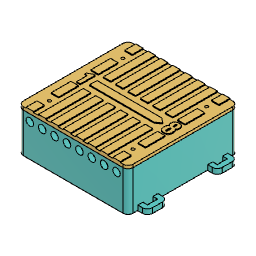
RelayBox (Autodesk Fusion 360 design; units mm, degrees)
Autodesk Fusion 360 part; units mm, degrees
(part 1 of 2)
sketch "Skizze1" plane through (0, 0, 0) normal (0, 0, 1) x (1, 0, 0)
  line L0 (0, 0) -> (110, 0)
  line L1 (110, 0) -> (110, 110)
  line L2 (110, 110) -> (0, 110)
  line L3 (0, 110) -> (0, 0)
  dimension "d1" = 110
  dimension "d2" = 110
  constraint horizontal L0
  constraint vertical L1
  constraint horizontal L2
  constraint vertical L3
  constraint coincident L0.start L3.end
  measures "d1" distance of L0.start L0.end
  measures "d2" distance of L0.start L2.end
extrude "Extrusion1" add sketch "Skizze1" along normal blind 40 makes body 1
sketch "Skizze2" plane through (0, 0, 0) normal (0, -1, 0) x (1, 0, 0)
  line L0 (0, 0) -> (110, 0)
  line L1 (110, 0) -> (110, 40)
  line L2 (110, 40) -> (0, 40)
  line L3 (0, 40) -> (0, 0)
  line L4 (0, 33) -> (110, 33)
  circle A0 centre (11.5, 33) radius 3.75
  circle A1 centre (11.5, 33) radius 5.5 construction
  circle A2 centre (-1832.7857, 33) radius 3.75
  circle A3 centre (-1832.7857, 33) radius 5.5 construction
  circle A4 centre (-3677.0714, 33) radius 3.75
  circle A5 centre (-3677.0714, 33) radius 5.5 construction
  circle A6 centre (-5521.3571, 33) radius 3.75
  circle A7 centre (-5521.3571, 33) radius 5.5 construction
  circle A8 centre (-7365.6429, 33) radius 3.75
  circle A9 centre (-7365.6429, 33) radius 5.5 construction
  circle A10 centre (-9209.9286, 33) radius 3.75
  circle A11 centre (-9209.9286, 33) radius 5.5 construction
  circle A12 centre (-11054.2143, 33) radius 3.75
  circle A13 centre (-11054.2143, 33) radius 5.5 construction
  circle A14 centre (-12898.5, 33) radius 3.75
  circle A15 centre (-12898.5, 33) radius 5.5 construction
  circle A16 centre (23.9286, 33) radius 5.5 construction
  circle A17 centre (23.9286, 33) radius 3.75
  circle A18 centre (36.3571, 33) radius 5.5 construction
  circle A19 centre (36.3571, 33) radius 3.75
  circle A20 centre (48.7857, 33) radius 5.5 construction
  circle A21 centre (48.7857, 33) radius 3.75
  circle A22 centre (61.2143, 33) radius 5.5 construction
  circle A23 centre (61.2143, 33) radius 3.75
  circle A24 centre (73.6429, 33) radius 5.5 construction
  circle A25 centre (73.6429, 33) radius 3.75
  circle A26 centre (86.0714, 33) radius 5.5 construction
  circle A27 centre (86.0714, 33) radius 3.75
  circle A28 centre (98.5, 33) radius 5.5 construction
  circle A29 centre (98.5, 33) radius 3.75
  dimension "d5" = 33
  dimension "d7" = 110
  dimension "d8" = 7.5
  dimension "d9" = 11.5
  dimension "d12" = 11
  dimension "d15" = -12910
  dimension "d16" = 0
  dimension "d19" = 87
  dimension "d20" = 0
  constraint coincident L3 L4.start
  constraint coincident L1 L4.end
  constraint perpendicular L1 L4
  constraint coincident L4 A0.centre
  constraint concentric A0 A1
  measures "d5" distance of L0 L4
  measures "d7" distance of L1.end L2.end
  measures "d8" diameter of A0
  measures "d9" distance of L3 A0.centre
  measures "d12" diameter of A1
extrude "Extrusion2" cut sketch "Skizze2" against normal blind 110 contours L4 A0 | L4 A0 | L4 A29 | L4 A29 | L4 A17 | L4 A17 | L4 A27 | L4 A27 | L4 A19 | L4 A19 | L4 A25 | L4 A25 | L4 A21 | L4 A21 | L4 A23 | L4 A23 bodies 1
sketch "Skizze3" plane through (0, 0, 40) normal (0, 0, 1) x (-1, 0, 0)
  line L0 (0, -110) -> (0, 0)
  line L1 (0, 0) -> (-110, 0)
  line L2 (-110, 0) -> (-110, -110)
  line L3 (-110, -110) -> (0, -110)
  line L4 (-105, -105) -> (-5, -105)
  line L5 (-5, -105) -> (-5, -5)
  line L6 (-5, -5) -> (-105, -5)
  line L7 (-105, -5) -> (-105, -105)
  dimension "d23" = -5
extrude "Extrusion3" cut sketch "Skizze3" against normal blind 35 contours L4 L5 L6 L7 bodies 1
sketch "Skizze4" plane through (0, 0, 5) normal (0, 0, 1) x (-1, 0, 0)
  line L0 (-105, -5) -> (-105, -105)
  line L1 (-105, -105) -> (-5, -105)
  line L2 (-5, -105) -> (-5, -5)
  line L3 (-5, -5) -> (-105, -5)
  line L4 (-100.75, -95.1) -> (-9.25, -95.1)
  line L5 (-9.25, -95.1) -> (-9.25, -14.9)
  line L6 (-9.25, -14.9) -> (-100.75, -14.9)
  line L7 (-100.75, -14.9) -> (-100.75, -95.1)
  dimension "d26" = 80.2
  dimension "d27" = 91.5
  dimension "d28" = 100
  dimension "d29" = 9.9
  dimension "d30" = 100
  dimension "d31" = 4.25
  constraint horizontal L4
  constraint vertical L5
  constraint horizontal L6
  constraint vertical L7
  measures "d26" distance of L4.start L6.end
  measures "d27" distance of L5.end L6.end
  measures "d28" distance of L1.end L2.end
  measures "d29" distance of L3 L6
  measures "d30" distance of L0.end L1.end
  measures "d31" distance of L0 L7
sketch "Skizze5" plane through (0, 0, 5) normal (0, 0, 1) x (-1, 0, 0)
  line L0 (-13.05, -18.1) -> (-13.05, -91.9)
  line L1 (-13.05, -91.9) -> (-96.95, -91.9)
  line L2 (-96.95, -91.9) -> (-96.95, -18.1)
  line L3 (-13.05, -18.1) -> (-96.95, -18.1)
  line L4 (0, 0) -> (-110, 0)
  line L5 (-5, -105) -> (-105, -105)
  line L6 (-105, -105) -> (-105, -5)
  line L7 (-105, -5) -> (-5, -5)
  line L8 (-5, -5) -> (-5, -105)
  line L9 (0, -110) -> (0, 0)
  line L10 (0, 0) -> (-110, 0)
  line L11 (-110, 0) -> (-110, -110)
  line L12 (-110, -110) -> (0, -110)
  line L13 (-55, 0) -> (-55, -110)
  line L14 (-110, -55) -> (0, -55)
  circle A0 centre (-96.95, -18.1) radius 2.5
  circle A1 centre (-96.95, -18.1) radius 5
  circle A2 centre (-13.05, -18.1) radius 2.5
  circle A3 centre (-13.05, -91.9) radius 2.5
  circle A4 centre (-96.95, -91.9) radius 2.5
  circle A5 centre (-96.95, -91.9) radius 5
  circle A6 centre (-13.05, -91.9) radius 5
  circle A7 centre (-13.05, -18.1) radius 5
  dimension "d32" = 73.8
  dimension "d33" = 83.9
  dimension "d34" = 73.8
  dimension "d35" = 5
  dimension "d36" = 10
  dimension "d37" = 5
  dimension "d38" = 5
  dimension "d39" = 5
  dimension "d40" = 10
  dimension "d41" = 10
  dimension "d42" = 10
  constraint vertical L0
  constraint perpendicular L0 L1
  constraint perpendicular L1 L2
  constraint midpoint L4 L13.start
  constraint midpoint L12 L13.end
  constraint midpoint L11 L14.start
  constraint midpoint L9 L14.end
  constraint symmetric L1 L3 L14
  constraint coincident L2.end L3.end
  constraint concentric A0 A1
  constraint coincident L0.start L3.start
  constraint coincident L0.end L1.start
  constraint coincident L1.end L2.start
  constraint concentric A4 A5
  constraint concentric A3 A6
  constraint concentric A2 A7
  measures "d32" distance of L0.start L0.end
  measures "d33" distance of L0.end L1.end
  measures "d34" distance of L1.end L2.end
  measures "d35" diameter of A0
  measures "d36" diameter of A1
  measures "d37" diameter of A2
  measures "d38" diameter of A3
  measures "d39" diameter of A4
  measures "d40" diameter of A5
  measures "d41" diameter of A6
  measures "d42" diameter of A7
extrude "Extrusion4" add sketch "Skizze5" along normal blind 3 contours L0 L3 A2 A7 | L0 L3 A2 A7 | L0 L1 A3 A6 | L0 L1 A3 A6 | L2 L3 A0 A1 | L2 L3 A0 A1 | L1 L2 A4 A5 | L1 L2 A4 A5 bodies 1
sketch "Skizze6" plane through (0, 0, 8) normal (0, 0, 1) x (-1, 0, 0)
  circle A0 centre (-96.95, -18.1) radius 2.5
  circle A1 centre (-96.95, -18.1) radius 5
  circle A2 centre (-96.95, -91.9) radius 2.5
  circle A3 centre (-96.95, -18.1) radius 2.5
  circle A4 centre (-13.05, -18.1) radius 2.5
  circle A5 centre (-13.05, -91.9) radius 2.5
  circle A6 centre (-13.05, -18.1) radius 2.5
extrude "Extrusion5" cut sketch "Skizze6" against normal blind 6 contours A0 A3 | A2 | A4 A6 | A5 bodies 1
sketch "Skizze7" plane through (0, 110, 0) normal (0, 1, 0) x (-1, 0, 0)
  circle A0 centre (-73.6429, 33) radius 3.75
  circle A1 centre (-23.9286, 33) radius 3.75
  circle A2 centre (-36.3571, 33) radius 3.75
  circle A3 centre (-86.0714, 33) radius 3.75
  circle A4 centre (-61.2143, 33) radius 3.75
  circle A5 centre (-11.5, 33) radius 3.75
  circle A6 centre (-48.7857, 33) radius 3.75
  circle A7 centre (-98.5, 33) radius 3.75
  line L0 (-110, 0) -> (0, 0)
  line L1 (0, 0) -> (0, 40)
  line L2 (0, 40) -> (-110, 40)
  line L3 (-110, 40) -> (-110, 0)
  line L4 (-99.45, 8) -> (-94.45, 8)
  line L5 (-15.55, 8) -> (-10.55, 8)
  line L6 (-94.45, 8) -> (-53.45, 8)
  line L7 (-15.55, 8) -> (-42.55, 8)
  line L8 (-53.45, 8) -> (-53.45, 14)
  line L9 (-42.55, 8) -> (-42.55, 14)
  line L10 (-42.55, 14) -> (-53.45, 14)
  line L11 (-53.45, 8) -> (-42.55, 8)
  dimension "d47" = 41
  dimension "d48" = 27
  dimension "d49" = 6
  dimension "d50" = 6
  constraint coincident L4.end L6.start
  constraint parallel L4 L6
  constraint coincident L5.start L7.start
  constraint parallel L5 L7
  constraint perpendicular L6 L8
  constraint perpendicular L7 L9
  measures "d47" distance of L4.end L6.end
  measures "d48" distance of L5.start L7.end
  measures "d49" distance of L6.end L8.end
  measures "d50" distance of L7.end L9.end
extrude "Extrusion6" cut sketch "Skizze7" against normal blind 5 contours L8 L9 L10 L11 bodies 1
sketch "Skizze8" plane through (0, 110, 0) normal (0, 1, 0) x (-1, 0, 0)
  line L0 (-42.55, 14) -> (-42.55, 8)
  line L1 (-42.55, 8) -> (-53.45, 8)
  line L2 (-53.45, 8) -> (-53.45, 14)
  line L3 (-53.45, 14) -> (-42.55, 14)
  circle A0 centre (-73.6429, 33) radius 3.75
  circle A1 centre (-23.9286, 33) radius 3.75
  circle A2 centre (-36.3571, 33) radius 3.75
  circle A3 centre (-86.0714, 33) radius 3.75
  circle A4 centre (-61.2143, 33) radius 3.75
  circle A5 centre (-11.5, 33) radius 3.75
  circle A6 centre (-48.7857, 33) radius 3.75
  circle A7 centre (-98.5, 33) radius 3.75
  line L4 (-110, 0) -> (0, 0)
  line L5 (0, 0) -> (0, 40)
  line L6 (0, 40) -> (-110, 40)
  line L7 (-110, 40) -> (-110, 0)
  circle A8 centre (-42.55, 11) radius 3
  circle A9 centre (-53.45, 11) radius 3
  constraint coincident L0.end A8
  constraint tangent L1 A8
  constraint coincident L0.start A8
  constraint coincident L1.end A9
  constraint tangent L1 A9
  constraint coincident L2.end A9
extrude "Extrusion7" cut sketch "Skizze8" against normal blind 5 contours L0 A8 | L2 A9 picked at (-41.5602, 11.1423) picked at (-54.4249, 10.7775) bodies 1
fillet "Abrundung1" radius 1 4 edges at (48, 110, 8) (56.45, 110, 11) (48, 110, 14) (39.55, 110, 11) on bodies 1
fillet "Abrundung2" radius 5 4 edges at (110, 110, 20) (110, 0, 20) (0, 0, 20) (0, 110, 20) on bodies 1
chamfer "Fase1" distance 0.4 angle 45 8 edges at (108.5355, 108.5355, 0) (55, 110, 0) (1.4645, 108.5355, 0) (0, 55, 0) (1.4645, 1.4645, 0) (55, 0, 0) (108.5355, 1.4645, 0) (110, 55, 0) on bodies 1
sketch "Skizze9" plane through (0, 0, 0) normal (0, 0, -1) x (1, 0, 0)
  arc A0 (105, -109.6) -> (109.6, -105) centre (105, -105) ccw
  line L0 (109.6, -105) -> (109.6, -5)
  arc A1 (109.6, -5) -> (105, -0.4) centre (105, -5) ccw
  line L1 (105, -0.4) -> (5, -0.4)
  arc A2 (5, -0.4) -> (0.4, -5) centre (5, -5) ccw
  line L2 (0.4, -5) -> (0.4, -105)
  arc A3 (0.4, -105) -> (5, -109.6) centre (5, -105) ccw
  line L3 (5, -109.6) -> (105, -109.6)
  line L4 (109.6, -95) -> (114.6, -95)
  line L5 (114.6, -95) -> (114.6, -85)
  line L6 (114.6, -85) -> (109.6, -85)
  line L7 (109.6, -85) -> (109.6, -95)
  line L8 (104.6, -100) -> (119.6, -100)
  line L9 (119.6, -100) -> (119.6, -80)
  line L10 (119.6, -80) -> (104.6, -80)
  line L11 (104.6, -80) -> (104.6, -100)
  line L12 (114.6, -15) -> (109.6, -15)
  line L13 (109.6, -15) -> (109.6, -25)
  line L14 (109.6, -25) -> (114.6, -25)
  line L15 (114.6, -25) -> (114.6, -15)
  line L16 (0.4, -15) -> (-4.6, -15)
  line L17 (-4.6, -15) -> (-4.6, -25)
  line L18 (-4.6, -25) -> (0.4, -25)
  line L19 (0.4, -25) -> (0.4, -15)
  line L20 (0.4, -85) -> (-4.6, -85)
  line L21 (-4.6, -85) -> (-4.6, -95)
  line L22 (-4.6, -95) -> (0.4, -95)
  line L23 (0.4, -95) -> (0.4, -85)
  line L24 (5, -110) -> (105, -110)
  line L25 (5.4, -100) -> (5.4, -80)
  line L26 (5.4, -80) -> (-9.6, -80)
  line L27 (-9.6, -80) -> (-9.6, -100)
  line L28 (-9.6, -100) -> (5.4, -100)
  line L29 (5.4, -30) -> (5.4, -10)
  line L30 (5.4, -10) -> (-9.6, -10)
  line L31 (-9.6, -10) -> (-9.6, -30)
  line L32 (-9.6, -30) -> (5.4, -30)
  line L33 (104.6, -30) -> (119.6, -30)
  line L34 (119.6, -30) -> (119.6, -10)
  line L35 (119.6, -10) -> (104.6, -10)
  line L36 (104.6, -10) -> (104.6, -30)
  line L37 (105, 0) -> (5, 0)
  dimension "d60" = 5
  dimension "d61" = 10
  dimension "d62" = 5
  dimension "d66" = 5
  dimension "d67" = 5
  dimension "d68" = 5
  dimension "d69" = 10
  dimension "d70" = 10
  dimension "d71" = 10
  dimension "d72" = 10
  dimension "d73" = 5
  dimension "d74" = 5
  dimension "d75" = 5
  dimension "d76" = 10
  dimension "d77" = 10
  dimension "d78" = 10
  constraint horizontal L4
  constraint vertical L5
  constraint horizontal L6
  constraint vertical L7
  constraint coincident L0 L4.start
  constraint horizontal L12
  constraint vertical L13
  constraint horizontal L14
  constraint vertical L15
  constraint horizontal L16
  constraint vertical L17
  constraint horizontal L18
  constraint vertical L19
  constraint horizontal L20
  constraint vertical L21
  constraint horizontal L22
  constraint vertical L23
  constraint collinear L2 L23
  constraint collinear L2 L19
  constraint collinear L0 L13
  constraint collinear L4 L22
  measures "d60" distance of L4.start L4.end
  measures "d61" distance of L4.start L6.end
  measures "d62" distance of L4
  measures "d66" distance of L21.end L22.end
  measures "d67" distance of L17.end L18.end
  measures "d68" distance of L13.end L14.end
  measures "d69" distance of L12.start L14.end
  measures "d70" distance of L16.end L17.end
  measures "d71" distance of L20.end L21.end
  measures "d72" distance of L8 L24
  measures "d75" distance of L14
  measures "d76" distance of L35 L37
  measures "d77" distance of L30 L37
  measures "d78" distance of L24 L28
extrude "Extrusion8" add sketch "Skizze9" against normal blind 5 contours L0 L4 L5 L6 L8 L9 L10 bodies 1
extrude "Extrusion9" add sketch "Skizze9" against normal blind 5 contours L2 L20 L21 L22 L26 L27 L28 | L0 L12 L14 L15 L33 L34 L35 | L2 L16 L17 L18 L30 L31 L32 bodies 1
fillet "Abrundung3" radius 5 8 edges at (119.6, 10, 2.5) (-9.6, 10, 2.5) (119.6, 30, 2.5) (119.6, 100, 2.5) (119.6, 80, 2.5) (-9.6, 30, 2.5) (-9.6, 80, 2.5) (-9.6, 100, 2.5) on bodies 1
sketch "Skizze10" plane through (0, 0, 40) normal (0, 0, 1) x (-1, 0, 0)
  arc A0 (-5, -110) -> (0, -105) centre (-5, -105) ccw
  line L0 (0, -105) -> (0, -5)
  arc A1 (0, -5) -> (-5, 0) centre (-5, -5) ccw
  line L1 (-5, 0) -> (-105, 0)
  arc A2 (-105, 0) -> (-110, -5) centre (-105, -5) ccw
  line L2 (-110, -5) -> (-110, -105)
  arc A3 (-110, -105) -> (-105, -110) centre (-105, -105) ccw
  line L3 (-105, -110) -> (-5, -110)
  line L4 (-5, -105) -> (-105, -105)
  line L5 (-105, -105) -> (-105, -5)
  line L6 (-105, -5) -> (-5, -5)
  line L7 (-5, -5) -> (-5, -105)
  circle A4 centre (-13.05, -91.9) radius 2.5
  circle A5 centre (-13.05, -18.1) radius 2.5
  circle A6 centre (-96.95, -18.1) radius 2.5
  circle A7 centre (-96.95, -91.9) radius 2.5
  circle A8 centre (-96.95, -18.1) radius 2.5
  line L8 (-104, -6) -> (-6, -6)
  line L9 (-6, -6) -> (-6, -104)
  line L10 (-6, -104) -> (-104, -104)
  line L11 (-104, -104) -> (-104, -6)
  circle A9 centre (-13.05, -91.9) radius 1.5
  circle A10 centre (-13.05, -18.1) radius 1.5
  circle A11 centre (-96.95, -18.1) radius 1.5
  circle A12 centre (-96.95, -91.9) radius 1.5
  dimension "d83" = 1
  dimension "d86" = 3
  dimension "d87" = 3
  dimension "d88" = 3
  dimension "d89" = 3
  constraint concentric A4 A9
  constraint concentric A5 A10
  constraint concentric A6 A11
  constraint concentric A7 A12
  measures "d86" diameter of A9
  measures "d87" diameter of A10
  measures "d88" diameter of A11
  measures "d89" diameter of A12
extrude "Extrusion11" add sketch "Skizze10" against normal blind 1 separate body contours A4 | A5 | A6 A8 | A7 | L8 L9 L10 L11 makes body 2
sketch "Skizze12" plane through (0, 0, 40) normal (0, 0, 1) x (-1, 0, 0)
extrude "Extrusion12" add sketch "Skizze10" along normal blind 3 separate body contours A0 L0 A1 L1 A2 L2 A3 L3 | L4 L5 L6 L7 | L8 L9 L10 L11 makes body 3
combine "Kombinieren1" operation add target body 2 tool bodies 3
sketch "Skizze13" plane through (0, 0, 43) normal (0, 0, 1) x (-1, 0, 0)
  circle A0 centre (-96.95, -18.1) radius 2.5
  circle A1 centre (-13.05, -91.9) radius 2.5
  circle A2 centre (-96.95, -91.9) radius 2.5
  circle A3 centre (-13.05, -18.1) radius 2.5
  line L0 (-105, -110) -> (-5, -110)
  arc A4 (-5, -110) -> (0, -105) centre (-5, -105) ccw
  line L1 (0, -105) -> (0, -5)
  arc A5 (0, -5) -> (-5, 0) centre (-5, -5) ccw
  line L2 (-5, 0) -> (-105, 0)
  arc A6 (-105, 0) -> (-110, -5) centre (-105, -5) ccw
  line L3 (-110, -5) -> (-110, -105)
  arc A7 (-110, -105) -> (-105, -110) centre (-105, -105) ccw
  line L4 (-15.25, 0) -> (-7.75, 0)
  line L5 (-27.6786, 0) -> (-20.1786, 0)
  line L6 (-40.1071, 0) -> (-32.6071, 0)
  line L7 (-52.5357, 0) -> (-45.0357, 0)
  line L8 (-64.9643, 0) -> (-57.4643, 0)
  line L9 (-77.3929, 0) -> (-69.8929, 0)
  line L10 (-89.8214, 0) -> (-82.3214, 0)
  line L11 (-102.25, 0) -> (-94.75, 0)
  line L12 (-7.75, 0) -> (-15.25, 0)
  line L13 (-15.25, 0) -> (-15.25, -110)
  line L14 (-15.25, -110) -> (-7.75, -110)
  line L15 (-7.75, -110) -> (-7.75, 0)
  line L16 (-20.1786, 0) -> (-27.6786, 0)
  line L17 (-27.6786, 0) -> (-27.6786, -110)
  line L18 (-27.6786, -110) -> (-20.1786, -110)
  line L19 (-20.1786, -110) -> (-20.1786, 0)
  line L20 (-32.6071, 0) -> (-40.1071, 0)
  line L21 (-40.1071, 0) -> (-40.1071, -110)
  line L22 (-40.1071, -110) -> (-32.6071, -110)
  line L23 (-32.6071, -110) -> (-32.6071, 0)
  line L24 (-45.0357, 0) -> (-52.5357, 0)
  line L25 (-52.5357, 0) -> (-52.5357, -110)
  line L26 (-52.5357, -110) -> (-45.0357, -110)
  line L27 (-45.0357, -110) -> (-45.0357, 0)
  line L28 (-57.4643, 0) -> (-64.9643, 0)
  line L29 (-64.9643, 0) -> (-64.9643, -110)
  line L30 (-64.9643, -110) -> (-57.4643, -110)
  line L31 (-57.4643, -110) -> (-57.4643, 0)
  line L32 (-69.8929, 0) -> (-77.3929, 0)
  line L33 (-77.3929, 0) -> (-77.3929, -110)
  line L34 (-77.3929, -110) -> (-69.8929, -110)
  line L35 (-69.8929, -110) -> (-69.8929, 0)
  line L36 (-82.3214, 0) -> (-89.8214, 0)
  line L37 (-89.8214, 0) -> (-89.8214, -110)
  line L38 (-89.8214, -110) -> (-82.3214, -110)
  line L39 (-82.3214, -110) -> (-82.3214, 0)
  line L40 (-94.75, 0) -> (-102.25, 0)
  line L41 (-102.25, 0) -> (-102.25, -110)
  line L42 (-102.25, -110) -> (-94.75, -110)
  line L43 (-94.75, -110) -> (-94.75, 0)
  constraint horizontal L12
  constraint vertical L13
  constraint horizontal L14
  constraint vertical L15
  constraint coincident L0 L13.end
  constraint coincident L4.end L12.start
  constraint horizontal L16
  constraint vertical L17
  constraint horizontal L18
  constraint vertical L19
  constraint coincident L0 L17.end
  constraint coincident L5.end L16.start
  constraint perpendicular L20 L21
  constraint parallel L20 L22
  constraint parallel L21 L23
  constraint coincident L6.start L20.end
  constraint perpendicular L17 L20
  constraint coincident L6.end L20.start
  constraint perpendicular L24 L25
  constraint parallel L24 L26
  constraint parallel L25 L27
  constraint coincident L7.start L24.end
  constraint perpendicular L23 L24
  constraint coincident L7.end L24.start
  constraint perpendicular L28 L29
  constraint parallel L28 L30
  constraint parallel L29 L31
  constraint coincident L8.start L28.end
  constraint perpendicular L27 L28
  constraint coincident L8.end L28.start
  constraint perpendicular L32 L33
  constraint parallel L32 L34
  constraint parallel L33 L35
  constraint coincident L9.start L32.end
  constraint perpendicular L31 L32
  constraint coincident L9.end L32.start
  constraint perpendicular L36 L37
  constraint parallel L36 L38
  constraint parallel L37 L39
  constraint coincident L10.start L36.end
  constraint perpendicular L35 L36
  constraint coincident L10.end L36.start
  constraint perpendicular L40 L41
  constraint parallel L40 L42
  constraint parallel L41 L43
  constraint coincident L11.start L40.end
  constraint perpendicular L39 L40
  constraint coincident L11.end L40.start
extrude "Extrusion13" add sketch "Skizze13" along normal blind 0.9 contours A0 A2 L0 L2 L11 L40 L41 L42 L43 | L0 L2 L10 L36 L37 L38 L39 | L0 L2 L9 L32 L33 L34 L35 | L0 L2 L8 L28 L29 L30 L31 | L0 L2 L7 L24 L25 L26 L27 | L0 L2 L6 L20 L21 L22 L23 | L0 L2 L5 L16 L17 L18 L19 | A1 A3 L0 L2 L4 L12 L13 L14 L15 bodies 2
sketch "Skizze14" plane through (0, 0, 43.9) normal (0, 0, 1) x (-1, 0, 0)
  line L0 (-15.25, -93.0874) -> (-15.25, -110)
  line L1 (-15.25, -110) -> (-7.75, -110)
  line L2 (-7.75, -110) -> (-7.75, 0)
  line L3 (-7.75, 0) -> (-15.25, 0)
  line L4 (-15.25, 0) -> (-15.25, -16.9126)
  arc A0 (-15.25, -19.2874) -> (-15.25, -16.9126) centre (-13.05, -18.1) ccw
  line L5 (-15.25, -19.2874) -> (-15.25, -90.7126)
  arc A1 (-15.25, -93.0874) -> (-15.25, -90.7126) centre (-13.05, -91.9) ccw
  line L6 (-20.1786, -110) -> (-20.1786, 0)
  line L7 (-89.8214, 0) -> (-89.8214, -110)
  line L8 (-20.1786, -10.9715) -> (-5.9214, -10.9715)
  line L9 (-5.9214, -10.9715) -> (-5.9214, -25.2285)
  line L10 (-5.9214, -25.2285) -> (-20.1786, -25.2285)
  line L11 (-20.1786, -25.2285) -> (-20.1786, -10.9715)
  line L12 (-20.1786, -10.9715) -> (-5.9214, -25.2285) construction
  line L13 (-5.9214, -10.9715) -> (-20.1786, -25.2285) construction
  line L14 (-5.9214, -10.9715) -> (-107.1918, -10.9715)
  line L15 (-5.9214, -25.2285) -> (-107.1184, -25.2285)
  line L16 (-94.75, -16.9126) -> (-94.75, 0)
  line L17 (-94.75, 0) -> (-102.25, 0)
  line L18 (-102.25, 0) -> (-102.25, -110)
  line L19 (-102.25, -110) -> (-94.75, -110)
  line L20 (-94.75, -110) -> (-94.75, -93.0874)
  arc A2 (-94.75, -90.7126) -> (-94.75, -93.0874) centre (-96.95, -91.9) ccw
  line L21 (-94.75, -90.7126) -> (-94.75, -19.2874)
  arc A3 (-94.75, -16.9126) -> (-94.75, -19.2874) centre (-96.95, -18.1) ccw
  line L22 (-7.75, -99.0285) -> (-102.25, -99.0285)
  line L23 (-102.25, -84.7715) -> (-7.75, -84.7715)
  point P0 (-13.05, -18.1)
  point P1 (-13.05, -91.9)
  dimension "d96" = 14.257
  dimension "d97" = 14.257
  dimension "d98" = 7.1285
  constraint horizontal L8
  constraint perpendicular L8 L9
  constraint parallel L8 L10
  constraint parallel L9 L11
  constraint coincident L12 P0
  constraint coincident L13 P0
  constraint coincident P0 A0.centre
  constraint perpendicular L9 L14
  constraint perpendicular L2 L15
  constraint coincident L2 L22.start
  constraint coincident L18 L22.end
  constraint perpendicular L18 L22
  constraint coincident L18 L23.start
  constraint coincident L2 L23.end
  constraint perpendicular L2 L23
  measures "d96" distance of L8.end L9.end
  measures "d97" distance of L22 L23
  measures "d98" distance of L22 P1
extrude "Extrusion14" cut sketch "Skizze14" against normal blind 0.9 contours L0 L2 L5 A1 L22 L23 | L2 L4 A0 L5 L8 L10 L14 L15 | L18 L20 A2 L21 L22 L23 | L14 L15 L16 L18 L21 A3 bodies 2
sketch "Skizze15" plane through (0, 0, 43.9) normal (0, 0, 1) x (-1, 0, 0)
  line L0 (-7.75, -25.2285) -> (-15.25, -25.2285)
  line L1 (-15.25, -25.2285) -> (-15.25, -84.7715)
  line L2 (-15.25, -84.7715) -> (-7.75, -84.7715)
  line L3 (-7.75, -84.7715) -> (-7.75, -25.2285)
  line L4 (-7.75, -25.2285) -> (-7.75, -84.7715)
  line L5 (-7.75, -84.7715) -> (-15.25, -84.7715)
  line L6 (-15.25, -84.7715) -> (-15.25, -25.2285)
  line L7 (-15.25, -25.2285) -> (-7.75, -25.2285)
  line L8 (-7.75, -10.9715) -> (-15.25, -10.9715)
  line L9 (-15.25, -10.9715) -> (-15.25, 0)
  line L10 (-15.25, 0) -> (-20.1786, 0)
  line L11 (-20.1786, 0) -> (-20.1786, -110)
  line L12 (-20.1786, -110) -> (-15.25, -110)
  line L13 (-15.25, -110) -> (-15.25, -99.0285)
  line L14 (-15.25, -99.0285) -> (-7.75, -99.0285)
  line L15 (-7.75, -99.0285) -> (-7.75, -110)
  line L16 (-7.75, -110) -> (-5, -110)
  arc A0 (-5, -110) -> (0, -105) centre (-5, -105) ccw
  line L17 (0, -105) -> (0, -5)
  arc A1 (0, -5) -> (-5, 0) centre (-5, -5) ccw
  line L18 (-5, 0) -> (-7.75, 0)
  line L19 (-7.75, 0) -> (-7.75, -10.9715)
  circle A2 centre (-13.05, -18.1) radius 2.5
  circle A3 centre (-13.05, -91.9) radius 2.5
  line L20 (-102.25, -84.7715) -> (-102.25, -25.2285)
  line L21 (-102.25, -25.2285) -> (-94.75, -25.2285)
  line L22 (-94.75, -25.2285) -> (-94.75, -84.7715)
  line L23 (-94.75, -84.7715) -> (-102.25, -84.7715)
  circle A4 centre (-96.95, -91.9) radius 2.5
  circle A5 centre (-96.95, -18.1) radius 2.5
  line L24 (-102.25, -99.0285) -> (-94.75, -99.0285)
  line L25 (-94.75, -99.0285) -> (-94.75, -110)
  line L26 (-94.75, -110) -> (-89.8214, -110)
  line L27 (-89.8214, -110) -> (-89.8214, 0)
  line L28 (-89.8214, 0) -> (-94.75, 0)
  line L29 (-94.75, 0) -> (-94.75, -10.9715)
  line L30 (-94.75, -10.9715) -> (-102.25, -10.9715)
  line L31 (-102.25, -10.9715) -> (-102.25, 0)
  line L32 (-102.25, 0) -> (-105, 0)
  arc A6 (-105, 0) -> (-110, -5) centre (-105, -5) ccw
  line L33 (-110, -5) -> (-110, -105)
  arc A7 (-110, -105) -> (-105, -110) centre (-105, -105) ccw
  line L34 (-105, -110) -> (-102.25, -110)
  line L35 (-102.25, -110) -> (-102.25, -99.0285)
  line L36 (-7.75, -55) -> (-102.25, -55)
  line L37 (-108.5309, -45) -> (-1.4691, -45)
  line L38 (-1.4691, -45) -> (-1.4691, -65)
  line L39 (-1.4691, -65) -> (-108.5309, -65)
  line L40 (-108.5309, -65) -> (-108.5309, -45)
  line L41 (-108.5309, -45) -> (-1.4691, -65) construction
  line L42 (-1.4691, -45) -> (-108.5309, -65) construction
  point P0 (-55, -55)
  dimension "d101" = 20
  constraint midpoint L4 L36.start
  constraint midpoint L20 L36.end
  constraint horizontal L37
  constraint perpendicular L37 L38
  constraint parallel L37 L39
  constraint parallel L38 L40
  constraint coincident L41 P0
  constraint coincident L42 P0
  constraint midpoint L36 P0
  measures "d101" distance of L37.end L38.end
extrude "Extrusion15" cut sketch "Skizze15" against normal blind 0.9 contours L1 L3 L4 L6 L36 L37 | L1 L3 L4 L6 L36 L39 | L11 L27 L36 L37 | L11 L27 L36 L39 | L20 L22 L36 L37 | L20 L22 L36 L39 bodies 2
sketch "Skizze16" plane through (0, 0, 43) normal (0, 0, 1) x (-1, 0, 0)
  line L0 (-102.25, -45) -> (-102.25, -25.2285)
  line L1 (-102.25, -25.2285) -> (-94.75, -25.2285)
  line L2 (-94.75, -25.2285) -> (-94.75, -45)
  line L3 (-94.75, -45) -> (-102.25, -45)
  circle A0 centre (-96.95, -18.1) radius 2.5
  circle A1 centre (-96.95, -91.9) radius 2.5
  line L4 (-102.25, -65) -> (-94.75, -65)
  line L5 (-94.75, -65) -> (-94.75, -84.7715)
  line L6 (-94.75, -84.7715) -> (-102.25, -84.7715)
  line L7 (-102.25, -84.7715) -> (-102.25, -65)
  line L8 (-7.75, -65) -> (-7.75, -84.7715)
  line L9 (-7.75, -84.7715) -> (-15.25, -84.7715)
  line L10 (-15.25, -84.7715) -> (-15.25, -65)
  line L11 (-15.25, -65) -> (-7.75, -65)
  line L12 (-7.75, -45) -> (-15.25, -45)
  line L13 (-15.25, -45) -> (-15.25, -25.2285)
  line L14 (-15.25, -25.2285) -> (-7.75, -25.2285)
  line L15 (-7.75, -25.2285) -> (-7.75, -45)
  line L16 (-7.75, -10.9715) -> (-15.25, -10.9715)
  line L17 (-15.25, -10.9715) -> (-15.25, 0)
  line L18 (-15.25, 0) -> (-20.1786, 0)
  line L19 (-20.1786, 0) -> (-20.1786, -45)
  line L20 (-20.1786, -45) -> (-27.6786, -45)
  line L21 (-27.6786, -45) -> (-27.6786, 0)
  line L22 (-27.6786, 0) -> (-32.6071, 0)
  line L23 (-32.6071, 0) -> (-32.6071, -45)
  line L24 (-32.6071, -45) -> (-40.1071, -45)
  line L25 (-40.1071, -45) -> (-40.1071, 0)
  line L26 (-40.1071, 0) -> (-45.0357, 0)
  line L27 (-45.0357, 0) -> (-45.0357, -45)
  line L28 (-45.0357, -45) -> (-52.5357, -45)
  line L29 (-52.5357, -45) -> (-52.5357, 0)
  line L30 (-52.5357, 0) -> (-57.4643, 0)
  line L31 (-57.4643, 0) -> (-57.4643, -45)
  line L32 (-57.4643, -45) -> (-64.9643, -45)
  line L33 (-64.9643, -45) -> (-64.9643, 0)
  line L34 (-64.9643, 0) -> (-69.8929, 0)
  line L35 (-69.8929, 0) -> (-69.8929, -45)
  line L36 (-69.8929, -45) -> (-77.3929, -45)
  line L37 (-77.3929, -45) -> (-77.3929, 0)
  line L38 (-77.3929, 0) -> (-82.3214, 0)
  line L39 (-82.3214, 0) -> (-82.3214, -45)
  line L40 (-82.3214, -45) -> (-89.8214, -45)
  line L41 (-89.8214, -45) -> (-89.8214, 0)
  line L42 (-89.8214, 0) -> (-94.75, 0)
  line L43 (-94.75, 0) -> (-94.75, -10.9715)
  line L44 (-94.75, -10.9715) -> (-102.25, -10.9715)
  line L45 (-102.25, -10.9715) -> (-102.25, 0)
  line L46 (-102.25, 0) -> (-105, 0)
  arc A2 (-105, 0) -> (-110, -5) centre (-105, -5) ccw
  line L47 (-110, -5) -> (-110, -105)
  arc A3 (-110, -105) -> (-105, -110) centre (-105, -105) ccw
  line L48 (-105, -110) -> (-102.25, -110)
  line L49 (-102.25, -110) -> (-102.25, -99.0285)
  line L50 (-102.25, -99.0285) -> (-94.75, -99.0285)
  line L51 (-94.75, -99.0285) -> (-94.75, -110)
  line L52 (-94.75, -110) -> (-89.8214, -110)
  line L53 (-89.8214, -110) -> (-89.8214, -65)
  line L54 (-89.8214, -65) -> (-82.3214, -65)
  line L55 (-82.3214, -65) -> (-82.3214, -110)
  line L56 (-82.3214, -110) -> (-77.3929, -110)
  line L57 (-77.3929, -110) -> (-77.3929, -65)
  line L58 (-77.3929, -65) -> (-69.8929, -65)
  line L59 (-69.8929, -65) -> (-69.8929, -110)
  line L60 (-69.8929, -110) -> (-64.9643, -110)
  line L61 (-64.9643, -110) -> (-64.9643, -65)
  line L62 (-64.9643, -65) -> (-57.4643, -65)
  line L63 (-57.4643, -65) -> (-57.4643, -110)
  line L64 (-57.4643, -110) -> (-52.5357, -110)
  line L65 (-52.5357, -110) -> (-52.5357, -65)
  line L66 (-52.5357, -65) -> (-45.0357, -65)
  line L67 (-45.0357, -65) -> (-45.0357, -110)
  line L68 (-45.0357, -110) -> (-40.1071, -110)
  line L69 (-40.1071, -110) -> (-40.1071, -65)
  line L70 (-40.1071, -65) -> (-32.6071, -65)
  line L71 (-32.6071, -65) -> (-32.6071, -110)
  line L72 (-32.6071, -110) -> (-27.6786, -110)
  line L73 (-27.6786, -110) -> (-27.6786, -65)
  line L74 (-27.6786, -65) -> (-20.1786, -65)
  line L75 (-20.1786, -65) -> (-20.1786, -110)
  line L76 (-20.1786, -110) -> (-15.25, -110)
  line L77 (-15.25, -110) -> (-15.25, -99.0285)
  line L78 (-15.25, -99.0285) -> (-7.75, -99.0285)
  line L79 (-7.75, -99.0285) -> (-7.75, -110)
  line L80 (-7.75, -110) -> (-5, -110)
  arc A4 (-5, -110) -> (0, -105) centre (-5, -105) ccw
  line L81 (0, -105) -> (0, -5)
  arc A5 (0, -5) -> (-5, 0) centre (-5, -5) ccw
  line L82 (-5, 0) -> (-7.75, 0)
  line L83 (-7.75, 0) -> (-7.75, -10.9715)
  circle A6 centre (-13.05, -18.1) radius 2.5
  circle A7 centre (-13.05, -91.9) radius 2.5
  line L84 (-17.7143, -45) -> (-5.2857, -45)
  line L85 (-5.2857, -45) -> (-5.2857, -65)
  line L86 (-5.2857, -65) -> (-17.7143, -65)
  line L87 (-17.7143, -65) -> (-17.7143, -45)
  line L88 (-30.1429, -65) -> (-30.1429, -45)
  line L89 (-17.7143, -65) -> (-30.1429, -65)
  line L90 (-17.7143, -45) -> (-17.7143, -65)
  line L91 (-30.1429, -45) -> (-17.7143, -45)
  line L92 (-42.5714, -65) -> (-42.5714, -45)
  line L93 (-30.1429, -65) -> (-42.5714, -65)
  line L94 (-30.1429, -45) -> (-30.1429, -65)
  line L95 (-42.5714, -45) -> (-30.1429, -45)
  line L96 (-55, -65) -> (-55, -45)
  line L97 (-42.5714, -65) -> (-55, -65)
  line L98 (-42.5714, -45) -> (-42.5714, -65)
  line L99 (-55, -45) -> (-42.5714, -45)
  line L100 (-67.4286, -65) -> (-67.4286, -45)
  line L101 (-55, -65) -> (-67.4286, -65)
  line L102 (-55, -45) -> (-55, -65)
  line L103 (-67.4286, -45) -> (-55, -45)
  line L104 (-79.8571, -65) -> (-79.8571, -45)
  line L105 (-67.4286, -65) -> (-79.8571, -65)
  line L106 (-67.4286, -45) -> (-67.4286, -65)
  line L107 (-79.8571, -45) -> (-67.4286, -45)
  line L108 (-92.2857, -65) -> (-92.2857, -45)
  line L109 (-79.8571, -65) -> (-92.2857, -65)
  line L110 (-79.8571, -45) -> (-79.8571, -65)
  line L111 (-92.2857, -45) -> (-79.8571, -45)
  line L112 (-104.7143, -65) -> (-104.7143, -45)
  line L113 (-92.2857, -65) -> (-104.7143, -65)
  line L114 (-92.2857, -45) -> (-92.2857, -65)
  line L115 (-104.7143, -45) -> (-92.2857, -45)
  line L116 (-5.2857, -45) -> (-17.7143, -45) construction
  line L117 (-17.7143, -45) -> (-17.7143, -65) construction
  line L118 (-17.7143, -65) -> (-5.2857, -65) construction
  line L119 (-5.2857, -65) -> (-5.2857, -45) construction
  line L120 (-92.2857, -45) -> (-104.7143, -45) construction
  line L121 (-104.7143, -45) -> (-104.7143, -65) construction
  line L122 (-104.7143, -65) -> (-92.2857, -65) construction
  line L123 (-92.2857, -65) -> (-92.2857, -45) construction
  dimension "d104" = 17.3571
  dimension "d105" = 4.9286
  dimension "d106" = 2.4643
  dimension "d107" = 2.4643
  dimension "d110" = -87
  dimension "d111" = 0
  dimension "d112" = 15
  dimension "d113" = 15
  text T0 "1" font "Impact" height 15 align centre middle in box 12.4286 x 20 at (-5.2857, -45) x (-1, 0) y (0, -1) spacing 1 kerned
  text T1 "8" font "Impact" height 15 align centre middle in box 12.4286 x 20 at (-92.2857, -45) x (-1, 0) y (0, -1) spacing 1 kerned
  constraint horizontal L84
  constraint vertical L85
  constraint horizontal L86
  constraint vertical L87
  constraint collinear L11 L86
  constraint collinear L20 L84
  constraint coincident L86.end
  constraint coincident L84.end
  constraint coincident L112.start
  constraint coincident L108.end
  measures "d104" distance of L12.end L23.end
  measures "d105" distance of L12.end L19.end
  measures "d106" distance of L13 L87
  measures "d107" distance of L15 L85
extrude "Extrusion16" add sketch "Skizze16" along normal blind 0.9 text T0 T1 bodies 2
sketch "Skizze17" plane through (0, 0, 43) normal (0, 0, 1) x (-1, 0, 0)
  spline S0 degree 3 poles (-101.2424, -56.0053) (-101.4993, -55.8834) (-101.9991, -55.6463) (-102.344, -55.2145) (-102.5117, -55.0046) knots 0 0 0 0 0.084034 0.16353 0.16353 0.16353 0.16353
  spline S1 degree 3 poles (-102.5117, -55.0046) (-102.6393, -54.6353) (-102.9898, -53.6205) (-102.9694, -52.5411) (-102.9565, -51.8545) knots 0 0 0 0 0.116519 0.320189 0.320189 0.320189 0.320189
  spline S2 degree 3 poles (-102.9565, -51.8545) (-102.9544, -51.3248) (-102.9508, -50.4155) (-102.7064, -49.5416) (-102.6044, -49.177) knots 0 0 0 0 0.157982 0.271128 0.271128 0.271128 0.271128
  spline S3 degree 3 poles (-102.6044, -49.177) (-102.45, -48.8976) (-102.1215, -48.3033) (-101.5409, -47.9478) (-101.2332, -47.7594) knots 0 0 0 0 0.094114 0.200246 0.200246 0.200246 0.200246
  spline S4 degree 3 poles (-101.2332, -47.7594) (-100.8403, -47.6004) (-99.9658, -47.2465) (-99.0206, -47.2247) (-98.5, -47.2128) knots 0 0 0 0 0.126135 0.28077 0.28077 0.28077 0.28077
  spline S5 degree 3 poles (-98.5, -47.2128) (-97.995, -47.2238) (-97.0815, -47.2438) (-96.2371, -47.5873) (-95.8595, -47.7409) knots 0 0 0 0 0.14998 0.271283 0.271283 0.271283 0.271283
  spline S6 degree 3 poles (-95.8595, -47.7409) (-95.5608, -47.9257) (-94.9838, -48.2827) (-94.6307, -48.861) (-94.4605, -49.1399) knots 0 0 0 0 0.103727 0.200337 0.200337 0.200337 0.200337
  spline S7 degree 3 poles (-94.4605, -49.1399) (-94.3399, -49.524) (-94.0444, -50.4652) (-94.0438, -51.4544) (-94.0435, -52.0398) knots 0 0 0 0 0.120183 0.294445 0.294445 0.294445 0.294445
  spline S8 degree 3 poles (-94.0435, -52.0398) (-94.0493, -52.4647) (-94.0601, -53.2574) (-94.188, -54.0395) (-94.2474, -54.4024) knots 0 0 0 0 0.127264 0.237425 0.237425 0.237425 0.237425
  spline S9 degree 3 poles (-94.2474, -54.4024) (-94.3653, -54.7245) (-94.6159, -55.4089) (-95.2352, -55.7988) (-95.563, -56.0053) knots 0 0 0 0 0.100073 0.212645 0.212645 0.212645 0.212645
  spline S10 degree 3 poles (-95.563, -56.0053) (-95.345, -56.134) (-94.904, -56.3945) (-94.6463, -56.8374) (-94.5161, -57.0615) knots 0 0 0 0 0.074612 0.15095 0.15095 0.15095 0.15095
  spline S11 degree 3 poles (-94.5161, -57.0615) (-94.4163, -57.3351) (-94.1984, -57.9326) (-94.1821, -58.5694) (-94.1733, -58.9145) knots 0 0 0 0 0.086816 0.189552 0.189552 0.189552 0.189552
  spline S12 degree 3 poles (-94.1733, -58.9145) (-94.2011, -59.503) (-94.2526, -60.5897) (-94.9351, -61.4294) (-95.248, -61.8144) knots 0 0 0 0 0.171436 0.316557 0.316557 0.316557 0.316557
  spline S13 degree 3 poles (-95.248, -61.8144) (-95.6821, -62.0973) (-96.6536, -62.7304) (-97.8186, -62.767) (-98.4629, -62.7872) knots 0 0 0 0 0.152673 0.341629 0.341629 0.341629 0.341629
  spline S14 degree 3 poles (-98.4629, -62.7872) (-99.1861, -62.7788) (-100.4361, -62.7643) (-101.4531, -62.0569) (-101.8817, -61.7588) knots 0 0 0 0 0.210731 0.364237 0.364237 0.364237 0.364237
  spline S15 degree 3 poles (-101.8817, -61.7588) (-102.1568, -61.3559) (-102.7586, -60.4744) (-102.8028, -59.4033) (-102.8267, -58.8218) knots 0 0 0 0 0.143562 0.314061 0.314061 0.314061 0.314061
  spline S16 degree 3 poles (-102.8267, -58.8218) (-102.8252, -58.4686) (-102.8225, -57.8643) (-102.603, -57.3037) (-102.5117, -57.0707) knots 0 0 0 0 0.104759 0.17925 0.17925 0.17925 0.17925
  spline S17 degree 3 poles (-102.5117, -57.0707) (-102.3638, -56.8823) (-102.0165, -56.4403) (-101.5247, -56.1639) (-101.2424, -56.0053) knots 0 0 0 0 0.07123 0.167142 0.167142 0.167142 0.167142
  line L0 (-14.664, -62.5) -> (-14.664, -47.5)
  line L1 (-14.664, -47.5) -> (-10.9209, -47.5)
  line L2 (-10.9209, -47.5) -> (-10.9209, -55.542)
  spline S18 degree 3 poles (-10.9209, -55.542) (-10.9254, -56.0074) (-10.9322, -56.7072) (-10.8613, -57.4029) (-10.8376, -57.6359) knots 0 0 0 0 0.139453 0.209683 0.209683 0.209683 0.209683
  spline S19 degree 3 poles (-10.8376, -57.6359) (-10.7949, -57.747) (-10.7058, -57.9792) (-10.4879, -58.1007) (-10.3743, -58.164) knots 0 0 0 0 0.034599 0.072268 0.072268 0.072268 0.072268
  spline S20 degree 3 poles (-10.3743, -58.164) (-10.1745, -58.2172) (-9.6299, -58.3621) (-9.0645, -58.3543) (-8.7066, -58.3493) knots 0 0 0 0 0.061805 0.168453 0.168453 0.168453 0.168453
  line L3 (-8.7066, -58.3493) -> (-8.336, -58.3493)
  line L4 (-8.336, -58.3493) -> (-8.336, -60.1004)
  spline S21 degree 3 poles (-8.336, -60.1004) (-9.1727, -60.3292) (-10.7638, -60.7644) (-11.9137, -61.9418) (-12.4589, -62.5) knots 0 0 0 0 0.254912 0.484769 0.484769 0.484769 0.484769
  line L5 (-12.4589, -62.5) -> (-14.664, -62.5)
  line L6 (-102.25, -45) -> (-102.25, -25.2285)
  line L7 (-102.25, -25.2285) -> (-94.75, -25.2285)
  line L8 (-94.75, -25.2285) -> (-94.75, -45)
  line L9 (-94.75, -45) -> (-102.25, -45)
  circle A0 centre (-96.95, -18.1) radius 2.5
  circle A1 centre (-96.95, -91.9) radius 2.5
  line L10 (-102.25, -65) -> (-94.75, -65)
  line L11 (-94.75, -65) -> (-94.75, -84.7715)
  line L12 (-94.75, -84.7715) -> (-102.25, -84.7715)
  line L13 (-102.25, -84.7715) -> (-102.25, -65)
  line L14 (-7.75, -65) -> (-7.75, -84.7715)
  line L15 (-7.75, -84.7715) -> (-15.25, -84.7715)
  line L16 (-15.25, -84.7715) -> (-15.25, -65)
  line L17 (-15.25, -65) -> (-7.75, -65)
  line L18 (-7.75, -45) -> (-15.25, -45)
  line L19 (-15.25, -45) -> (-15.25, -25.2285)
  line L20 (-15.25, -25.2285) -> (-7.75, -25.2285)
  line L21 (-7.75, -25.2285) -> (-7.75, -45)
  line L22 (-7.75, -10.9715) -> (-15.25, -10.9715)
  line L23 (-15.25, -10.9715) -> (-15.25, 0)
  line L24 (-15.25, 0) -> (-20.1786, 0)
  line L25 (-20.1786, 0) -> (-20.1786, -45)
  line L26 (-20.1786, -45) -> (-27.6786, -45)
  line L27 (-27.6786, -45) -> (-27.6786, 0)
  line L28 (-27.6786, 0) -> (-32.6071, 0)
  line L29 (-32.6071, 0) -> (-32.6071, -45)
  line L30 (-32.6071, -45) -> (-40.1071, -45)
  line L31 (-40.1071, -45) -> (-40.1071, 0)
  line L32 (-40.1071, 0) -> (-45.0357, 0)
  line L33 (-45.0357, 0) -> (-45.0357, -45)
  line L34 (-45.0357, -45) -> (-52.5357, -45)
  line L35 (-52.5357, -45) -> (-52.5357, 0)
  line L36 (-52.5357, 0) -> (-57.4643, 0)
  line L37 (-57.4643, 0) -> (-57.4643, -45)
  line L38 (-57.4643, -45) -> (-64.9643, -45)
  line L39 (-64.9643, -45) -> (-64.9643, 0)
  line L40 (-64.9643, 0) -> (-69.8929, 0)
  line L41 (-69.8929, 0) -> (-69.8929, -45)
  line L42 (-69.8929, -45) -> (-77.3929, -45)
  line L43 (-77.3929, -45) -> (-77.3929, 0)
  line L44 (-77.3929, 0) -> (-82.3214, 0)
  line L45 (-82.3214, 0) -> (-82.3214, -45)
  line L46 (-82.3214, -45) -> (-89.8214, -45)
  line L47 (-89.8214, -45) -> (-89.8214, 0)
  line L48 (-89.8214, 0) -> (-94.75, 0)
  line L49 (-94.75, 0) -> (-94.75, -10.9715)
  line L50 (-94.75, -10.9715) -> (-102.25, -10.9715)
  line L51 (-102.25, -10.9715) -> (-102.25, 0)
  line L52 (-102.25, 0) -> (-105, 0)
  arc A2 (-105, 0) -> (-110, -5) centre (-105, -5) ccw
  line L53 (-110, -5) -> (-110, -105)
  arc A3 (-110, -105) -> (-105, -110) centre (-105, -105) ccw
  line L54 (-105, -110) -> (-102.25, -110)
  line L55 (-102.25, -110) -> (-102.25, -99.0285)
  line L56 (-102.25, -99.0285) -> (-94.75, -99.0285)
  line L57 (-94.75, -99.0285) -> (-94.75, -110)
  line L58 (-94.75, -110) -> (-89.8214, -110)
  line L59 (-89.8214, -110) -> (-89.8214, -65)
  line L60 (-89.8214, -65) -> (-82.3214, -65)
  line L61 (-82.3214, -65) -> (-82.3214, -110)
  line L62 (-82.3214, -110) -> (-77.3929, -110)
  line L63 (-77.3929, -110) -> (-77.3929, -65)
  line L64 (-77.3929, -65) -> (-69.8929, -65)
  line L65 (-69.8929, -65) -> (-69.8929, -110)
  line L66 (-69.8929, -110) -> (-64.9643, -110)
  line L67 (-64.9643, -110) -> (-64.9643, -65)
  line L68 (-64.9643, -65) -> (-57.4643, -65)
  line L69 (-57.4643, -65) -> (-57.4643, -110)
  line L70 (-57.4643, -110) -> (-52.5357, -110)
  line L71 (-52.5357, -110) -> (-52.5357, -65)
  line L72 (-52.5357, -65) -> (-45.0357, -65)
  line L73 (-45.0357, -65) -> (-45.0357, -110)
  line L74 (-45.0357, -110) -> (-40.1071, -110)
  line L75 (-40.1071, -110) -> (-40.1071, -65)
  line L76 (-40.1071, -65) -> (-32.6071, -65)
  line L77 (-32.6071, -65) -> (-32.6071, -110)
  line L78 (-32.6071, -110) -> (-27.6786, -110)
  line L79 (-27.6786, -110) -> (-27.6786, -65)
  line L80 (-27.6786, -65) -> (-20.1786, -65)
  line L81 (-20.1786, -65) -> (-20.1786, -110)
  line L82 (-20.1786, -110) -> (-15.25, -110)
  line L83 (-15.25, -110) -> (-15.25, -99.0285)
  line L84 (-15.25, -99.0285) -> (-7.75, -99.0285)
  line L85 (-7.75, -99.0285) -> (-7.75, -110)
  line L86 (-7.75, -110) -> (-5, -110)
  arc A4 (-5, -110) -> (0, -105) centre (-5, -105) ccw
  line L87 (0, -105) -> (0, -5)
  arc A5 (0, -5) -> (-5, 0) centre (-5, -5) ccw
  line L88 (-5, 0) -> (-7.75, 0)
  line L89 (-7.75, 0) -> (-7.75, -10.9715)
  circle A6 centre (-13.05, -18.1) radius 2.5
  circle A7 centre (-13.05, -91.9) radius 2.5
  line L90 (-20.1786, -65) -> (-20.1786, -45)
  line L91 (-89.8214, -45) -> (-89.8214, -65)
  line L92 (-89.8214, -55) -> (-20.1786, -55)
  line L93 (-77.3929, -45) -> (-89.8214, -55)
  line L94 (-89.8214, -55) -> (-77.3929, -65)
  line L95 (-77.3929, -45) -> (-77.3929, -65)
  line L96 (-20.1786, -58.75) -> (-85.1607, -58.75)
  line L97 (-20.1786, -51.25) -> (-85.1607, -51.25)
  dimension "d116" = 3.75
  dimension "d117" = 3.75
  constraint coincident L80.end L81.start
  constraint coincident L25.end L26.start
  constraint coincident L46.end L47.start
  constraint coincident L59.end L60.start
  constraint midpoint L91 L92.start
  constraint midpoint L90 L92.end
  constraint coincident L42.end L43.start
  constraint coincident L63.end L64.start
  constraint coincident L90 L96.start
  constraint coincident L94 L96.end
  constraint perpendicular L90 L96
  constraint coincident L90 L97.start
  constraint parallel L96 L97
  constraint coincident L93 L97.end
  measures "d116" distance of L92 L96
  measures "d117" distance of L92 L97
extrude "Extrusion17" add sketch "Skizze17" along normal blind 0.9 contours L90 L92 L95 L97 | L90 L92 L95 L96 | L92 L93 L95 L97 | L92 L94 L95 L96 bodies 2
ref_plane "Arbeitsebene1" through (55, 55, 40) normal (0, 0, -1) x (1, 0, 0)
split "Teilen1" by plane through (55, 55, 40) normal (0, 0, -1) bodies 2 makes body 4 at (68.5758, 43.0614, 39)